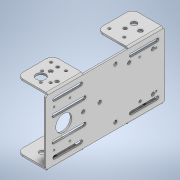
# Autodesk Inventor part: podstawa
Saved by Autodesk Inventor 2022 (Build 260153000, 153)
## iProperties
Created: 2025-04-22
Part Number: podstawa
Material: Ogólny
Document SubType Name: Modeling
Designer: Olga Kowalczyk IB 240875
Density: 1 g/cm^3
Appearance: Domyślna
Author: Olga Kowalczyk IB 240875
Autodesk Inventor part; units mm, degrees
ref_plane "YZ Plane" through (0, 0, 0) normal (1, 0, 0) x (0, 1, 0)
sketch "Szkic1" plane through (0, 0, 0) normal (1, 0, 0) x (0, 1, 0)
  line L0 (2, 0) -> (73, 0)
  line L1 (75, -2) -> (75, -137.5)
  line L2 (73, -139.5) -> (2, -139.5)
  line L3 (0, -137.5) -> (0, -2)
  arc A0 (75, -2) -> (73, 0) centre (73, -2) ccw
  arc A1 (0, -137.5) -> (2, -139.5) centre (2, -137.5) ccw
  arc A2 (2, 0) -> (0, -2) centre (2, -2) ccw
  arc A3 (73, -139.5) -> (75, -137.5) centre (73, -137.5) ccw
  line L4 (75, -2) -> (77, -2)
  line L5 (77, -2) -> (77, -43.5)
  line L6 (77, -43.5) -> (75, -43.5)
  line L7 (37.5, 0) -> (37.5, -139.5)
  line L8 (75, -69.75) -> (0, -69.75)
  line L9 (0, -2) -> (-2, -2)
  line L10 (-2, -2) -> (-2, -43.5)
  line L11 (-2, -43.5) -> (0, -43.5)
  line L12 (0, -69.75) -> (75, -69.75) construction
  line L13 (75, -137.5) -> (77, -137.5)
  line L14 (77, -137.5) -> (77, -96)
  line L15 (77, -96) -> (75, -96)
  line L16 (-2, -137.5) -> (-2, -96)
  line L17 (-2, -96) -> (0, -96)
  line L18 (0, -137.5) -> (-2, -137.5)
  circle A4 centre (37.5, -20.95) radius 9.5
  circle A5 centre (37.5, -43.5) radius 2
  circle A6 centre (37.5, -63) radius 2
  arc A7 (53, -9) -> (49, -9) centre (51, -9) ccw
  arc A8 (49, -45) -> (53, -45) centre (51, -45) ccw
  arc A9 (69, -10) -> (65, -10) centre (67, -10) ccw
  arc A10 (65, -41) -> (69, -41) centre (67, -41) ccw
  line L19 (69, -10) -> (69, -41)
  line L20 (65, -41) -> (65, -10)
  line L21 (53, -9) -> (53, -45)
  line L22 (49, -45) -> (49, -9)
  circle A11 centre (59.5, -9.5) radius 1
  circle A12 centre (59.5, -28) radius 1
  circle A13 centre (67, -81.5) radius 2
  arc A14 (69, -100) -> (65, -100) centre (67, -100) ccw
  arc A15 (65, -130.5) -> (69, -130.5) centre (67, -130.5) ccw
  line L23 (69, -100) -> (69, -130.5)
  line L24 (65, -130.5) -> (65, -100)
  circle A16 centre (60.5, -125.5) radius 2
  circle A17 centre (59.5, -129.5) radius 1
  arc A18 (26, -9) -> (22, -9) centre (24, -9) ccw
  arc A19 (22, -45) -> (26, -45) centre (24, -45) ccw
  arc A20 (10, -10) -> (6, -10) centre (8, -10) ccw
  arc A21 (6, -41) -> (10, -41) centre (8, -41) ccw
  line L25 (6, -10) -> (6, -41)
  line L26 (10, -41) -> (10, -10)
  line L27 (22, -9) -> (22, -45)
  line L28 (26, -45) -> (26, -9)
  circle A22 centre (15.5, -9.5) radius 1
  circle A23 centre (15.5, -28) radius 1
  circle A24 centre (8, -81.5) radius 2
  arc A25 (10, -100) -> (6, -100) centre (8, -100) ccw
  arc A26 (6, -130.5) -> (10, -130.5) centre (8, -130.5) ccw
  line L29 (6, -100) -> (6, -130.5)
  line L30 (10, -130.5) -> (10, -100)
  circle A27 centre (14.5, -125.5) radius 2
  circle A28 centre (15.5, -129.5) radius 1
  circle A29 centre (60.5, -97.5) radius 2
  circle A30 centre (60, -110) radius 1
  circle A31 centre (14.5, -110.5) radius 1.5
  point P0 (0, 0)
  point P1 (75, 0)
  point P2 (75, -139.5)
  point P3 (37.5, -69.75)
  point P4 (2, -2)
  point P5 (2, -137.5)
  point P6 (0, -96)
  dimension "d0" = 75
  dimension "d1" = 139.5
  dimension "d2" = 2
  dimension "d3" = 2
  dimension "d4" = 2
  dimension "d5" = 2
  dimension "d6" = 2
  dimension "d7" = 41.5
  dimension "d8" = 19
  dimension "d9" = 4
  dimension "d10" = 4
  dimension "d11" = 63
  dimension "d12" = 43.5
  dimension "d13" = 20.95
  dimension "d14" = 4
  dimension "d15" = 4
  dimension "d16" = 4
  dimension "d17" = 4
  dimension "d18" = 10
  dimension "d19" = 9
  dimension "d20" = 41
  dimension "d21" = 45
  dimension "d22" = 8
  dimension "d23" = 24
  dimension "d24" = 2
  dimension "d25" = 2
  dimension "d26" = 7.5
  dimension "d28" = 9.5
  dimension "d29" = 18.5
  dimension "d30" = 4
  dimension "d31" = 4
  dimension "d32" = 4
  dimension "d33" = 9
  dimension "d34" = 39.5
  dimension "d35" = 58
  dimension "d36" = 4
  dimension "d37" = 2
  dimension "d38" = 14
  dimension "d39" = 10
  dimension "d45" = 4.5
  dimension "d46" = 5.5
  dimension "d47" = 4
  dimension "d48" = 2
  dimension "d49" = 3
  dimension "d50" = 29
  dimension "d51" = 42
  dimension "d52" = 29.5
  dimension "d53" = 5
  constraints: 62 end point, 40 symmetric about line, 32 centre point, 32 point on circle, 20 tangent, 10 point on line, 8 coincident, 8 vertical alignment, 5 midpoint, 5 perpendicular, 2 horizontal, 11 other
  measures "d0" distance of point (0, 0) point (75, 0)
  measures "d1" distance of point (75, 0) point (75, -139.5)
  measures "d2" radius of A0
  measures "d3" radius of A1
  measures "d4" radius of A2
  measures "d5" radius of A3
  measures "d6" distance of L1.start L4.end
  measures "d7" distance of L4.end L5.end
  measures "d8" diameter of A4
  measures "d9" diameter of A5
  measures "d10" diameter of A6
  measures "d11" distance of L7.start A6.centre
  measures "d12" distance of L7.start A5.centre
  measures "d13" distance of L7.start A4.centre
  measures "d14" diameter of A7
  measures "d15" diameter of A8
  measures "d16" diameter of A9
  measures "d17" diameter of A10
  measures "d18" distance from line of L0 A9.centre
  measures "d19" distance from line of L0 A7.centre
  measures "d20" distance from line of L0 A10.centre
  measures "d21" distance from line of L0 A8.centre
  measures "d22" distance from line of L1 A9.centre
  measures "d23" distance from line of L1 A7.centre
  measures "d24" diameter of A11
  measures "d25" diameter of A12
  measures "d26" horizontal distance of A9.centre A11.centre
  measures "d28" distance from line of L0 A11.centre
  measures "d29" distance of A11.centre A12.centre
  measures "d30" diameter of A13
  measures "d31" diameter of A14
  measures "d32" diameter of A15
  measures "d33" distance from line of L2 A15.centre
  measures "d34" distance from line of L2 A14.centre
  measures "d35" distance from line of L2 A13.centre
  measures "d36" diameter of A16
  measures "d37" diameter of A17
  measures "d38" distance from line of L2 A16.centre
  measures "d39" distance from line of L2 A17.centre
  measures "d45" distance from line of L24 A16.centre
  measures "d46" distance from line of L24 A17.centre
  measures "d47" diameter of A29
  measures "d48" diameter of A30
  measures "d49" diameter of A31
  measures "d50" distance from line of L2 A31.centre
  measures "d51" distance from line of L2 A29.centre
  measures "d52" distance from line of L2 A30.centre
  measures "d53" distance from line of L24 A30.centre
extrude "Wyciągnięcie proste1" add sketch "Szkic1" along normal blind 2 contours L0 L7 A4 A5 A6 L8 L3 A2 | L0 A0 L1 L8 L7 A6 A5 A4 | L8 L7 L2 A1 L3 | L8 L1 A3 L2 L7
extrude "Wyciągnięcie proste2" add sketch "Szkic1" along normal blind 2 and the other way blind 34 contours L3 L11 L10 L9 | L4 L5 L6 L1 | L3 L18 L16 L17 | L15 L14 L13 L1
fillet "Zaokrąglenie1" radius 7 8 edges at (-34, 76, -2) (-34, 76, -43.5) (-34, 76, -137.5) (-34, 76, -96) (-34, -1, -137.5) (-34, -1, -96) (-34, -1, -43.5) (-34, -1, -2)
fillet "Zaokrąglenie2" radius 2 4 edges at (2, -2, -116.75) (2, -2, -22.75) (2, 77, -116.75) (2, 77, -22.75)
fillet "Zaokrąglenie3" radius 0.5 4 edges at (0, 75, -22.75) (0, 75, -116.75) (0, 0, -22.75) (0, 0, -116.75)
ref_plane "Płaszczyzna konstrukcyjna1" through (-27, -2, -137.5) normal (0, -1, 0) x (1, 0, 0)
sketch "Szkic2" plane through (-27, -2, -137.5) normal (0, -1, 0) x (1, 0, 0)
  circle A0 centre (8, 13) radius 5.5
  circle A1 centre (20, 12.5) radius 1.5
  circle A2 centre (14, 7) radius 1.5
  circle A3 centre (22.5, 17.5) radius 2
  circle A4 centre (8.5, 24) radius 2.25
  circle A5 centre (3, 19.5) radius 1.5
  circle A6 centre (-3.5, 12.5) radius 1.5
  circle A7 centre (17, 33.5) radius 1.5
  circle A8 centre (8.25, 32.5) radius 1.75
  circle A9 centre (-0.5, 33.5) radius 1.5
  circle A10 centre (17, 102) radius 1.5
  circle A11 centre (-0.5, 102) radius 1.5
  circle A12 centre (8.5, 111.5) radius 2
  circle A13 centre (22, 118) radius 2.5
  circle A14 centre (8.75, 121.75) radius 3.25
  line L0 (-7, 7) -> (-7, 34.5) projected
  line L1 (27, 0) -> (0, 0) projected
  line L2 (0, 41.5) -> (27, 41.5) projected
  line L3 (0, 135.5) -> (27, 135.5) projected
  line L4 (27, 94) -> (0, 94) projected
  line L5 (-7, 101) -> (-7, 128.5) projected
  line L6 (29, 94) -> (29, 135.5) projected
  point P0 (27, 137.5)
  dimension "d63" = 11
  dimension "d64" = 3
  dimension "d65" = 3
  dimension "d66" = 4
  dimension "d67" = 4.5
  dimension "d68" = 3
  dimension "d69" = 3
  dimension "d70" = 3
  dimension "d71" = 3.5
  dimension "d72" = 3
  dimension "d73" = 3
  dimension "d74" = 3
  dimension "d75" = 4
  dimension "d76" = 5
  dimension "d77" = 6.5
  dimension "d78" = 6.5
  dimension "d79" = 15.25
  dimension "d80" = 24
  dimension "d81" = 15.5
  dimension "d82" = 29.5
  dimension "d83" = 10
  dimension "d84" = 27
  dimension "d85" = 21
  dimension "d86" = 3.5
  dimension "d87" = 15
  dimension "d88" = 17.5
  dimension "d89" = 12.5
  dimension "d90" = 7
  dimension "d91" = 13
  dimension "d92" = 12.5
  dimension "d93" = 19.5
  dimension "d94" = 8
  dimension "d95" = 9
  dimension "d96" = 17.5
  dimension "d97" = 17.5
  dimension "d98" = 13.75
  dimension "d99" = 8
  dimension "d100" = 17.5
  dimension "d101" = 15.75
  dimension "d102" = 7
  dimension "d103" = 15.5
  dimension "d104" = 6.5
  dimension "d105" = 24
  constraints: 15 centre point, 2 horizontal alignment
  measures "d63" diameter of A0
  measures "d64" diameter of A1
  measures "d65" diameter of A2
  measures "d66" diameter of A3
  measures "d67" diameter of A4
  measures "d68" diameter of A5
  measures "d69" diameter of A6
  measures "d70" diameter of A7
  measures "d71" diameter of A8
  measures "d72" diameter of A9
  measures "d73" diameter of A10
  measures "d74" diameter of A11
  measures "d75" diameter of A12
  measures "d76" diameter of A13
  measures "d77" diameter of A14
  measures "d78" distance from line of L0 A9.centre
  measures "d79" distance from line of L0 A8.centre
  measures "d80" distance from line of L0 A7.centre
  measures "d81" distance from line of L0 A4.centre
  measures "d82" distance from line of L0 A3.centre
  measures "d83" distance from line of L0 A5.centre
  measures "d84" distance from line of L0 A1.centre
  measures "d85" distance from line of L0 A2.centre
  measures "d86" distance from line of L0 A6.centre
  measures "d87" distance from line of L0 A0.centre
  measures "d88" distance from line of L1 A3.centre
  measures "d89" distance from line of L1 A1.centre
  measures "d90" distance from line of L1 A2.centre
  measures "d91" distance from line of L1 A0.centre
  measures "d92" distance from line of L1 A6.centre
  measures "d93" distance from line of L1 A5.centre
  measures "d94" distance from line of L2 A9.centre
  measures "d95" distance from line of L2 A8.centre
  measures "d96" distance from line of L2 A4.centre
  measures "d97" distance from line of L3 A13.centre
  measures "d98" distance from line of L3 A14.centre
  measures "d99" distance from line of L4 A10.centre
  measures "d100" distance from line of L4 A12.centre
  measures "d101" distance from line of L5 A14.centre
  measures "d102" distance from line of L6 A13.centre
  measures "d103" distance from line of L5 A12.centre
  measures "d104" distance from line of L5 A11.centre
  measures "d105" distance from line of L5 A10.centre
extrude "Wyciągnięcie proste3" cut sketch "Szkic2" against normal blind 2
ref_plane "Płaszczyzna konstrukcyjna7" through (0, 77, -137.5) normal (0, 1, 0) x (1, 0, 0)
sketch "Szkic6" plane through (0, 77, -137.5) normal (0, 1, 0) x (1, 0, 0)
  circle A0 centre (-19, -122.5) radius 5.5
  circle A1 centre (-7, -123) radius 1.5
  circle A2 centre (-13, -128.5) radius 1.5
  circle A3 centre (-4.5, -118) radius 2
  circle A4 centre (-18.5, -111.5) radius 2.25
  circle A5 centre (-24, -116) radius 1.5
  circle A6 centre (-30.5, -123) radius 1.5
  circle A7 centre (-10, -102) radius 1.5
  circle A8 centre (-18.75, -103) radius 1.75
  circle A9 centre (-27.5, -102) radius 1.5
  circle A10 centre (-10, -33.5) radius 1.5
  circle A11 centre (-27.5, -33.5) radius 1.5
  circle A12 centre (-18.5, -24) radius 2
  circle A13 centre (-7, -17.5) radius 2.5
  circle A14 centre (-18.25, -13.75) radius 3.25
  line L0 (-34, -128.5) -> (-34, -101)
  line L1 (0, -135.5) -> (-27, -135.5)
  line L2 (-27, -94) -> (0, -94)
  line L3 (0, 0) -> (0, 0)
  line L4 (0, -41.5) -> (-27, -41.5)
  line L5 (-34, -34.5) -> (-34, -7)
  line L6 (0, -41.5) -> (0, 0)
  point P0 (0, -137.5)
  point P1 (0, 2)
  point P2 (-27, -135.5)
  point P3 (0, 2)
  dimension "d109" = 11
  dimension "d110" = 3
  dimension "d111" = 3
  dimension "d112" = 4
  dimension "d113" = 4.5
  dimension "d114" = 3
  dimension "d115" = 3
  dimension "d116" = 3
  dimension "d117" = 3.5
  dimension "d118" = 3
  dimension "d119" = 3
  dimension "d120" = 3
  dimension "d121" = 4
  dimension "d122" = 5
  dimension "d123" = 6.5
  dimension "d124" = 6.5
  dimension "d125" = 15.25
  dimension "d126" = 24
  dimension "d127" = 15.5
  dimension "d128" = 29.5
  dimension "d129" = 10
  dimension "d130" = 27
  dimension "d131" = 21
  dimension "d132" = 3.5
  dimension "d133" = 15
  dimension "d134" = 17.5
  dimension "d135" = 12.5
  dimension "d136" = 7
  dimension "d137" = 13
  dimension "d138" = 12.5
  dimension "d139" = 19.5
  dimension "d140" = 8
  dimension "d141" = 9
  dimension "d142" = 17.5
  dimension "d143" = 17.5
  dimension "d144" = 13.75
  dimension "d145" = 8
  dimension "d146" = 17.5
  dimension "d147" = 15.75
  dimension "d148" = 7
  dimension "d149" = 15.5
  dimension "d150" = 6.5
  dimension "d151" = 24
  dimension "d152" = 2
  dimension "d153" = 34
  dimension "d154" = 0
  constraints: 15 centre point, 14 end point, 12 coincident, 2 horizontal alignment, 1 parallel
  measures "d109" diameter of A0
  measures "d110" diameter of A1
  measures "d111" diameter of A2
  measures "d112" diameter of A3
  measures "d113" diameter of A4
  measures "d114" diameter of A5
  measures "d115" diameter of A6
  measures "d116" diameter of A7
  measures "d117" diameter of A8
  measures "d118" diameter of A9
  measures "d119" diameter of A10
  measures "d120" diameter of A11
  measures "d121" diameter of A12
  measures "d122" diameter of A13
  measures "d123" diameter of A14
  measures "d124" distance from line of L0 A9.centre
  measures "d125" distance from line of L0 A8.centre
  measures "d126" distance from line of L0 A7.centre
  measures "d127" distance from line of L0 A4.centre
  measures "d128" distance from line of L0 A3.centre
  measures "d129" distance from line of L0 A5.centre
  measures "d130" distance from line of L0 A1.centre
  measures "d131" distance from line of L0 A2.centre
  measures "d132" distance from line of L0 A6.centre
  measures "d133" distance from line of L0 A0.centre
  measures "d134" distance from line of L1 A3.centre
  measures "d135" distance from line of L1 A1.centre
  measures "d136" distance from line of L1 A2.centre
  measures "d137" distance from line of L1 A0.centre
  measures "d138" distance from line of L1 A6.centre
  measures "d139" distance from line of L1 A5.centre
  measures "d140" distance from line of L2 A9.centre
  measures "d141" distance from line of L2 A8.centre
  measures "d142" distance from line of L2 A4.centre
  measures "d143" distance from line of L3 A13.centre
  measures "d144" distance from line of L3 A14.centre
  measures "d145" distance from line of L4 A10.centre
  measures "d146" distance from line of L4 A12.centre
  measures "d147" distance from line of L5 A14.centre
  measures "d148" distance from line of L6 A13.centre
  measures "d149" distance from line of L5 A12.centre
  measures "d150" distance from line of L5 A11.centre
  measures "d151" distance from line of L5 A10.centre
  measures "d152" distance of point (0, 0) point (0, 2)
  measures "d153" distance from line of L5 point (0, 2)
  measures "d154" distance from line of L3.start L6
extrude "Wyciągnięcie proste4" cut sketch "Szkic6" against normal blind 2 contours A0 | A1 | A2 | A3 | A4 | A5 | A7 | A8 | A9 | A10 | A11 | A12 | A13 | A14
